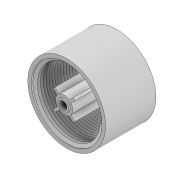
# Autodesk Inventor part: PMCover
Saved by Autodesk Inventor 2020 (Build 240168000, 168)
## iProperties
Created: 2020-05-07
Part Number: PMCover
Material: Generic
Document SubType Name: Modeling
Designer: Theo Cominotto
Density: 1 g/cm^3
Appearance: Default
Author: Theo Cominotto
Autodesk Inventor part; units mm, degrees
ref_plane "YZ Plane" through (0, 0, 0) normal (1, 0, 0) x (0, 1, 0)
ref_plane "XZ Plane" through (0, 0, 0) normal (0, 1, 0) x (-1, 0, 0)
sketch "Sketch1" plane through (0, 0, 0) normal (0, 0, 1) x (1, 0, 0)
  circle A0 centre (0, 0) radius 17
  circle A1 centre (0, 0) radius 15.4
  dimension "d1" = 30.8
  dimension "d2" = 1.6
  constraints: 2 centre point, 2 coincident
  measures "d1" diameter of A1
  measures "d2" radial gap between concentric circles of A0 A1
extrude "Extrusion1" add sketch "Sketch1" along normal blind 20
sketch "Sketch2" plane through (0, 0, 0) normal (0, 0, -1) x (-1, 0, 0)
  circle A0 centre (0, 0) radius 17 projected
  line L0 (0, 0) -> (0, 8) construction
  circle A1 centre (0, 8) radius 4
  circle A2 centre (-8, 0) radius 4
  circle A3 centre (0, -8) radius 4
  circle A4 centre (8, 0) radius 4
  circle A5 centre (0, 0) radius 1.75
  dimension "d5" = 8
  dimension "d6" = 8
  dimension "d9" = 360
  dimension "d11" = 3.5
  constraints: 5 centre point, 2 coincident, 2 end point, 1 vertical, 9 other
  measures "d5" distance of L0.start L0.end
  measures "d6" diameter of A1
  measures "d11" diameter of A5
extrude "Extrusion2" add sketch "Sketch2" along normal blind 2
sketch "Sketch3" plane through (0, 0, 0) normal (0, 0, 1) x (1, 0, 0)
  circle A0 centre (0, 0) radius 1.75 projected
  circle A1 centre (0, 0) radius 3.75
  line L0 (-4.7518, 3.9669) -> (3.9669, -4.7518)
  line L1 (3.9669, -4.7518) -> (4.7518, -3.9669)
  line L2 (4.7518, -3.9669) -> (-3.9669, 4.7518)
  line L3 (-3.9669, 4.7518) -> (-4.7518, 3.9669)
  line L4 (-4.7518, 3.9669) -> (4.7518, -3.9669) construction
  line L5 (3.9669, -4.7518) -> (-3.9669, 4.7518) construction
  line L6 (0, -23.8) -> (0, 23.8) construction
  line L7 (-23.8, 0) -> (23.8, 0) construction
  line L8 (-4.7518, -3.9669) -> (3.9669, 4.7518)
  line L9 (3.9669, 4.7518) -> (4.7518, 3.9669)
  line L10 (4.7518, 3.9669) -> (-3.9669, -4.7518)
  line L11 (-3.9669, -4.7518) -> (-4.7518, -3.9669)
  line L12 (-4.7518, -3.9669) -> (4.7518, 3.9669) construction
  line L13 (3.9669, 4.7518) -> (-3.9669, -4.7518) construction
  point P0 (-3.0149, 2.23)
  point P1 (-3.0149, -2.23)
  point P2 (-2.23, -3.0149)
  point P3 (2.23, -3.0149)
  point P4 (3.0149, -2.23)
  point P5 (3.0149, 2.23)
  point P6 (2.23, 3.0149)
  point P7 (-2.23, 3.0149)
  dimension "d14" = 7.5
  dimension "d15" = 1.11
  dimension "d16" = 45
  dimension "d17" = 1.11
  dimension "d18" = 45
  dimension "d19" = 12.33
  dimension "d20" = 12.33
  constraints: 24 end point, 4 midpoint, 4 parallel, 2 perpendicular, 1 centre point, 1 coincident
  measures "d14" diameter of A1
  measures "d15" distance of L1.end L0.end
  measures "d16" angle of L6 L0
  measures "d17" distance of L8.end L9.end
  measures "d18" angle of L6 L8
  measures "d19" distance between parallel lines of L3 L1
  measures "d20" distance between parallel lines of L9 L11
extrude "Extrusion3" add sketch "Sketch3" along normal blind 21.11 contours A0 L10 A1 L2 | A0 L8 A1 L10 | L2 A1 L0 A0 | A0 L2 A1 L8 | A1 L8 L9 L10 | L0 A1 L10 A0 | L2 L1 L0 A1 | A0 L0 A1 L2 | L10 A1 L8 A0 | A0 L8 A1 L0 | A1 L0 L3 L2 | L10 L11 L8 A1
sketch "Sketch4" plane through (0, 0, 0) normal (0, 1, 0) x (-1, 0, 0)
  line L0 (-15.4, 20) -> (15.4, 20) projected
  line L1 (-15.4, 20) -> (-15.4, 0) projected
  line L2 (-15.4, 20) -> (-14, 19.375)
  line L3 (-14, 19.375) -> (-15.4, 18.75)
  line L4 (-15.4, 20) -> (-15.4, 0) projected
  line L5 (-14, 19.375) -> (-15.4, 19.375) construction
  line L6 (-15.4, 20) -> (-15.4, 0) construction
  point P0 (0, 0)
  dimension "d54" = 1.4
  dimension "d55" = 1.25
  constraints: 6 end point, 2 point on line, 1 perpendicular, 1 other
  measures "d54" distance from line of L1 L2.end
  measures "d55" distance of L3.end L1.start
ref_plane "Work Plane1" through (0, 0, 19.1) normal (0, 0, 1) x (1, 0, 0)
sketch "Sketch6" plane through (0, 0, 21.11) normal (0, 0, 1) x (1, 0, 0)
  circle A0 centre (0, 0) radius 2.65
  circle A1 centre (0, 0) radius 1.75 projected
  dimension "d51" = 5.3
  constraints: 1 centre point, 1 coincident
  measures "d51" diameter of A0
extrude "Extrusion4" add sketch "Sketch6" along normal blind 0.5
coil "Coil3" sketch "Sketch4" operation add axis through (0, 0, -10) along (0, 0, -1) pitch 1.25 turns 16 hand right
chamfer "Chamfer1" distance 0.559 angle 45 2 edges at (14.7, 0, 19.6875) (14.7, 0, 19.0625)
equation "\"d17\" = d15"
equation "\"d20\" = d19"
equation "\"d54\" = ThreadHeight"
equation "\"d55\" = ThreadPitch"
equation "\"d56\" = ThreadPitch"
equation "\"ThreadTol\" = 0.8"
equation "\"ThreadHeight\" = 1.4"
equation "\"ThreadPitch\" = 1.25"
body "Solid1"
